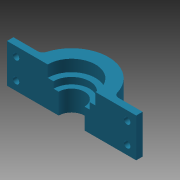
# Autodesk Inventor part: 砂轮架带动曲轴固定盖
Saved by Autodesk Inventor 2015 (Build 190159000, 159)
## iProperties
Created: 2017-05-17
Part Number: 砂轮架带动曲轴固定盖
Material: 常规
Document SubType Name: Modeling
Designer: Administrator
Density: 1 g/cm^3
Appearance: 青绿色
Author: Administrator
Autodesk Inventor part; units mm, degrees
ref_plane "YZ Plane" through (0, 0, 0) normal (1, 0, 0) x (0, 1, 0)
ref_plane "XZ Plane" through (0, 0, 0) normal (0, 1, 0) x (-1, 0, 0)
ref_plane "XY Plane" through (0, 0, 0) normal (0, 0, 1) x (1, 0, 0)
sketch "草图1" plane through (0, 0, 0) normal (0, 0, 1) x (1, 0, 0)
  arc A0 (28.5, 0) -> (-28.5, 0) centre (0, 0) ccw
  line L0 (-50, 0) -> (50, 0)
  line L1 (50, 0) -> (50, 5)
  line L2 (50, 5) -> (-50, 5)
  line L3 (-50, 5) -> (-50, 0)
  dimension "d0" = 57
  dimension "d1" = 100
  dimension "d2" = 5
  constraints: 8 end point, 2 coincident, 2 parallel, 2 point on circle, 2 point on line, 1 centre point, 1 horizontal, 1 midpoint, 1 perpendicular
  measures "d0" diameter of A0
  measures "d1" distance of L2.end L1.end
  measures "d2" distance of L2.end L0.start
extrude "拉伸1" add sketch "草图1" along normal blind 30
sketch "草图2" plane through (0, 0, 30) normal (0, 0, 1) x (1, 0, 0)
  circle A0 centre (0, 0) radius 18.5
  dimension "d5" = 37
  constraints: 1 centre point, 1 coincident
  measures "d5" diameter of A0
extrude "拉伸2" cut sketch "草图2" against normal blind 9
sketch "草图3" plane through (0, 0, 21) normal (0, 0, 1) x (1, 0, 0)
  circle A0 centre (0, 0) radius 14
  dimension "d8" = 28
  constraints: 1 centre point, 1 coincident
  measures "d8" diameter of A0
extrude "拉伸3" cut sketch "草图3" against normal blind 5
sketch "草图4" plane through (0, 0, 16) normal (0, 0, 1) x (1, 0, 0)
  circle A0 centre (0, 0) radius 10
  dimension "d11" = 20
  constraints: 1 centre point, 1 coincident
  measures "d11" diameter of A0
extrude "拉伸4" cut sketch "草图4" against normal through all
fillet "圆角1" radius 4 2 edges at (28.058, 5, 15) (-28.058, 5, 15)
sketch "草图5" plane through (50, 5, 30) normal (0, 1, 0) x (1, 0, 0)
  circle A0 centre (-7, 23) radius 2.5
  circle A1 centre (-7, 7) radius 2.5
  circle A2 centre (-93, 7) radius 2.5
  circle A3 centre (-93, 23) radius 2.5
  line L0 (-81.229, 30) -> (-100, 30) projected
  line L1 (-100, 30) -> (-100, 0) projected
  line L2 (-81.229, 0) -> (-100, 0) projected
  line L3 (0, 30) -> (-18.771, 30) projected
  line L4 (0, 30) -> (0, 0) projected
  line L5 (0, 0) -> (-18.771, 0) projected
  point P0 (-50, 30)
  dimension "d15" = 5
  dimension "d16" = 5
  dimension "d17" = 5
  dimension "d18" = 5
  dimension "d19" = 7
  dimension "d20" = 7
  dimension "d21" = 7
  dimension "d22" = 7
  dimension "d23" = 7
  dimension "d24" = 7
  dimension "d25" = 7
  dimension "d26" = 7
  constraints: 4 centre point
  measures "d15" diameter of A0
  measures "d16" diameter of A1
  measures "d17" diameter of A2
  measures "d18" diameter of A3
  measures "d19" distance from line of L0 A3.centre
  measures "d20" distance from line of L1 A3.centre
  measures "d21" distance from line of A2.centre L1
  measures "d22" distance from line of L2 A2.centre
  measures "d23" distance from line of L3 A0.centre
  measures "d24" distance from line of L4 A0.centre
  measures "d25" distance from line of L4 A1.centre
  measures "d26" distance from line of L5 A1.centre
extrude "拉伸5" cut sketch "草图5" against normal through all
